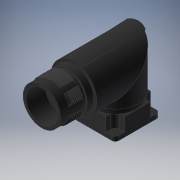
# Autodesk Inventor part: Connector-41,4D-c
Saved by Autodesk Inventor 2019 (Build 230136000, 136)
## iProperties
Created: 2024-01-27
Part Number: Connector-41,4D-c
Material: Generic
Catalog Web Link: www.cadenas.de
Description: AKM2G_CON1-Connector
Vendor: KOLLMORGEN
Document SubType Name: Modeling
Designer: psAdmin
Manufacturer: KOLLMORGEN
Mass: 32.2721 g
Surface Area: 81.4823 cm^2
Volume: 32.2721 cm^3
Density: 1 g/cm^3
Appearance: PSOLRGB-175-175-175
Category: PARTsolutions
Company: KOLLMORGEN
Title: Connector-41,4D-c
Author: Cadenas PARTsolutions
Comments: Connector
PSOL_IDENT_0: {$CADENAS_DATA/23d-libs/kollmorgen/akm2g/parts/akm2g_connector1.prj},181 {VTYP=3D},{NB=Connector-41,
PSOL_IDENT_1: 4D-c},{LINA=Connector-41,4D-c},{NN=AKM2G_CON1},{DATE=22.01.2022 17:38:51},{GEOMDATE=12.11.2021 08:57
PSOL_IDENT_2: :11},{VERSION=},{LINEID=10},{WBVAR=CON},{WBNUMERIC=}  {NB=Connector-41,4D-c},{LINA=Connector-41,4D-c
PSOL_IDENT_3: },{KT=DUMMY},{PN=Connector-41,4},{CON=D}
NB: Connector-41,4D-c
NN: AKM2G_CON1
NT: Connector
NBSYN: $PN.$CON.-c
LINA: Connector-41,4D-c
CATALOG: Kollmorgen
PN: Connector-41,4
CON: Single right angle M23
SUPPLIER: KOLLMORGEN
ARTICLENO: Connector-41,4D-c
BOMINFO: Connector-41,4D-c
CREATOR: CADENAS GmbH
Autodesk Inventor part; units mm, degrees
sketch "Sketch20" plane through (0, 29, 0) normal (0, 1, 0) x (-1, 0, 0)
  line L0 (-28.35, -66.0503) -> (-28.35, -87.7503)
  arc A0 (-28.35, -87.7503) -> (-26.35, -89.7503) centre (-26.35, -87.7503) ccw
  line L1 (-26.35, -89.7503) -> (-4.65, -89.7503)
  arc A1 (-4.65, -89.7503) -> (-2.65, -87.7503) centre (-4.65, -87.7503) ccw
  line L2 (-2.65, -87.7503) -> (-2.65, -66.0503)
  arc A2 (-2.65, -66.0503) -> (-4.65, -64.0503) centre (-4.65, -66.0503) ccw
  line L3 (-4.65, -64.0503) -> (-26.35, -64.0503)
  arc A3 (-26.35, -64.0503) -> (-28.35, -66.0503) centre (-26.35, -66.0503) ccw
  constraints: 8 end point, 8 point on circle, 4 centre point
extrude "Extrusion1" add sketch "Sketch20" along normal blind 10.2
sketch "Sketch21" plane through (0, 39.2, 0) normal (0, 1, 0) x (1, 0, 0)
  line L0 (-101.9389, -26.7472) -> (82.9421, -26.7472)
  line L1 (82.9421, -26.7472) -> (82.9421, 149.7843)
  line L2 (82.9421, 149.7843) -> (-101.9389, 149.7843)
  line L3 (-101.9389, 149.7843) -> (-101.9389, -26.7472)
  line L4 (-50, 69.5009) -> (5.6005, 69.5009)
  arc A0 (8.1005, 67.0009) -> (5.6005, 69.5009) centre (5.6005, 67.0009) ccw
  line L5 (8.1005, 67.0009) -> (8.1005, 0)
  line L6 (8.1005, 0) -> (22.8995, 0)
  line L7 (22.8995, 0) -> (22.8995, 67.0009)
  arc A1 (25.3995, 69.5009) -> (22.8995, 67.0009) centre (25.3995, 67.0009) ccw
  line L8 (25.3995, 69.5009) -> (50, 69.5009)
  line L9 (50, 69.5009) -> (50, 84.2998)
  line L10 (50, 84.2998) -> (25.3995, 84.2998)
  arc A2 (22.8995, 86.7998) -> (25.3995, 84.2998) centre (25.3995, 86.7998) ccw
  line L11 (22.8995, 86.7998) -> (22.8995, 100)
  line L12 (22.8995, 100) -> (8.1005, 100)
  line L13 (8.1005, 100) -> (8.1005, 86.7998)
  arc A3 (5.6005, 84.2998) -> (8.1005, 86.7998) centre (5.6005, 86.7998) ccw
  line L14 (5.6005, 84.2998) -> (-50, 84.2998)
  line L15 (-50, 84.2998) -> (-50, 69.5009)
  constraints: 32 end point, 8 point on circle, 4 centre point
extrude "Extrusion2" cut sketch "Sketch21" against normal blind 7.7
sketch "Sketch22" plane through (15.5, 0, 0) normal (1, 0, 0) x (0, 0, -1)
  line L0 (76.9003, 65.3381) -> (76.9003, 39.2)
  line L1 (76.9003, 39.2) -> (64.4003, 39.2)
  line L2 (64.4003, 39.2) -> (64.4003, 41.9)
  line L3 (64.4003, 41.9) -> (64.8403, 41.9)
  line L4 (64.8403, 41.9) -> (64.8403, 42.2)
  line L5 (64.8403, 42.2) -> (63.6753, 42.2)
  line L6 (63.6753, 42.2) -> (63.6753, 55.45)
  line L7 (63.6753, 55.45) -> (76.9003, 55.45)
  line L8 (76.9003, 55.45) -> (76.9003, 39.2)
  constraints: 18 end point
revolve "Revolution1" add sketch "Sketch22" angle 360 about axis through (15.5, 65.3381, -76.9003) along (0, 1, 0)
sketch "Sketch23" plane through (15.5, 0, 0) normal (1, 0, 0) x (0, 0, -1)
  line L0 (90.1253, 55.45) -> (45.5003, 55.45)
  line L1 (45.5003, 55.45) -> (45.5003, 64.55)
  line L2 (45.5003, 64.55) -> (34.5003, 64.55)
  line L3 (34.5003, 64.55) -> (34.5003, 66.25)
  line L4 (34.5003, 66.25) -> (39.5003, 66.25)
  line L5 (39.5003, 66.25) -> (40.7128, 66.95)
  line L6 (40.7128, 66.95) -> (41.2499, 66.25)
  line L7 (41.2499, 66.25) -> (41.787, 66.95)
  line L8 (41.787, 66.95) -> (42.3242, 66.25)
  line L9 (42.3242, 66.25) -> (42.8613, 66.95)
  line L10 (42.8613, 66.95) -> (43.3984, 66.25)
  line L11 (43.3984, 66.25) -> (43.9356, 66.95)
  line L12 (43.9356, 66.95) -> (44.4727, 66.25)
  line L13 (44.4727, 66.25) -> (45.0098, 66.95)
  line L14 (45.0098, 66.95) -> (45.5469, 66.25)
  line L15 (45.5469, 66.25) -> (46.0841, 66.95)
  line L16 (46.0841, 66.95) -> (46.6212, 66.25)
  line L17 (46.6212, 66.25) -> (47.1583, 66.95)
  line L18 (47.1583, 66.95) -> (47.7003, 66.95)
  line L19 (47.7003, 66.95) -> (47.7003, 66.025)
  line L20 (47.7003, 66.025) -> (49.2003, 66.025)
  line L21 (49.2003, 66.025) -> (49.2003, 66.95)
  line L22 (49.2003, 66.95) -> (53.0003, 66.95)
  line L23 (53.0003, 66.95) -> (53.0003, 68.65)
  line L24 (53.0003, 68.65) -> (90.1253, 68.65)
  line L25 (90.1253, 68.65) -> (90.1253, 55.45)
  line L26 (90.1253, 55.45) -> (45.5003, 55.45)
  constraints: 54 end point
revolve "Revolution2" add sketch "Sketch23" angle 360 about axis through (15.5, 55.45, -90.1253) along (0, 0, -1)
sketch "Sketch24" plane through (15.5, 0, 0) normal (1, 0, 0) x (0, 0, -1)
  line L0 (96.8276, 55.45) -> (34.5003, 55.45)
  line L1 (53.0003, 69) -> (53.0003, 68)
  line L2 (53.0003, 68) -> (90.1253, 68)
  line L3 (90.1253, 68) -> (90.1253, 70.4)
  line L4 (90.1253, 70.4) -> (53.0003, 69)
  constraints: 10 end point
revolve "Revolution3" add sketch "Sketch24" angle 40 mid plane about axis through (15.5, 55.45, -96.8276) along (0, 0, 1)
sketch "Sketch25" plane through (0, 39.2, 0) normal (0, 1, 0) x (1, 0, 0)
  line L0 (2.275, 91.1253) -> (2.275, 76.9003)
  arc A0 (28.725, 76.9003) -> (2.275, 76.9003) centre (15.5, 76.9003) ccw
  line L1 (28.725, 76.9003) -> (28.725, 91.1253)
  line L2 (28.725, 91.1253) -> (2.275, 91.1253)
  constraints: 6 end point, 2 point on circle, 1 centre point
extrude "Extrusion3" cut sketch "Sketch25" along normal blind 40
sketch "Sketch26" plane through (0, 0, -34.5003) normal (0, 0, 1) x (1, 0, 0)
  line L0 (-5.9182, 26.0713) -> (32.7889, 26.0713)
  line L1 (32.7889, 26.0713) -> (32.7889, 78.1206)
  line L2 (32.7889, 78.1206) -> (-5.9182, 78.1206)
  line L3 (-5.9182, 78.1206) -> (-5.9182, 26.0713)
  arc A0 (4.9933, 57.95) -> (4.9933, 52.95) centre (15.5, 55.45) ccw
  line L4 (4.9933, 52.95) -> (4.9933, 40.1811)
  line L5 (4.9933, 40.1811) -> (16.5, 30.5923)
  line L6 (16.5, 30.5923) -> (16.5, 44.6964)
  arc A1 (16.5, 44.6964) -> (20.0643, 45.6619) centre (15.5, 55.45) ccw
  line L7 (20.0643, 45.6619) -> (26.0067, 32.9184)
  line L8 (26.0067, 32.9184) -> (26.0067, 52.95)
  arc A2 (26.0067, 52.95) -> (26.0067, 57.95) centre (15.5, 55.45) ccw
  line L9 (26.0067, 57.95) -> (26.0067, 65.9567)
  line L10 (26.0067, 65.9567) -> (23.1368, 63.0868)
  arc A3 (23.1368, 63.0868) -> (21, 64.7446) centre (15.5, 55.45) ccw
  line L11 (21, 64.7446) -> (21, 74.8152)
  line L12 (21, 74.8152) -> (8.75, 74.125)
  line L13 (8.75, 74.125) -> (8.75, 63.8807)
  arc A4 (8.75, 63.8807) -> (6.6532, 61.6446) centre (15.5, 55.45) ccw
  line L14 (6.6532, 61.6446) -> (4.9933, 62.8068)
  line L15 (4.9933, 62.8068) -> (4.9933, 57.95)
  constraints: 32 end point, 10 point on circle, 5 centre point
extrude "Extrusion4" cut sketch "Sketch26" against normal blind 13.2
ref_plane "to_XY" through (15.5, 29, -76.9003) normal (0, 1, 0) x (-1, 0, 0)
ref_plane "to_YZ" through (15.5, 29, -76.9003) normal (-1, 0, 0) x (0, 0, 1)
ref_plane "to_ZX" through (15.5, 29, -76.9003) normal (0, 0, 1) x (0, 1, 0)
body "Solid1"
